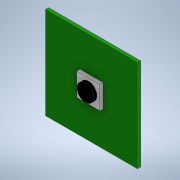
# Autodesk Inventor part: Nav_Camera
Saved by Autodesk Inventor 2020 (Build 240168000, 168)
## iProperties
Created: 2022-01-28
Part Number: Nav_Camera
Material: Generic
Document SubType Name: Modeling
Designer: danie
Density: 1 g/cm^3
Appearance: Default
Author: danie
Autodesk Inventor part; units mm, degrees
ref_plane "YZ Plane" through (0, 0, 0) normal (1, 0, 0) x (0, 1, 0)
ref_plane "XZ Plane" through (0, 0, 0) normal (0, 1, 0) x (-1, 0, 0)
ref_plane "XY Plane" through (0, 0, 0) normal (0, 0, 1) x (1, 0, 0)
sketch "Sketch1" plane through (0, 0, 0) normal (0, 0, 1) x (1, 0, 0)
  line L0 (0, 0) -> (38, 0)
  line L1 (38, 0) -> (38, -38)
  line L2 (38, -38) -> (0, -38)
  line L3 (0, -38) -> (0, 0)
  dimension "d0" = 38
  dimension "d1" = 38
  constraints: 8 end point, 2 parallel, 1 horizontal, 1 perpendicular
  measures "d0" distance of L1.end L2.end
  measures "d1" distance of L0.end L1.end
extrude "Extrusion1" add sketch "Sketch1" along normal blind 1.27
sketch "Sketch2" plane through (0, 0, 1.27) normal (0, 0, 1) x (1, 0, 0)
  line L0 (0, -38) -> (38, -38) construction
  line L1 (0, 0) -> (38, -38) construction
  line L2 (38, -38) -> (38, 0) construction
  line L3 (38, 0) -> (0, -38) construction
  line L4 (14.2571, -14.2571) -> (23.7429, -14.2571)
  line L5 (23.7429, -14.2571) -> (23.7429, -23.7429)
  line L6 (23.7429, -23.7429) -> (14.2571, -23.7429)
  line L7 (14.2571, -23.7429) -> (14.2571, -14.2571)
  line L8 (14.2571, -14.2571) -> (23.7429, -23.7429) construction
  line L9 (23.7429, -14.2571) -> (14.2571, -23.7429) construction
  point P0 (19, -19)
  constraints: 16 end point, 3 midpoint, 2 parallel, 1 horizontal, 1 perpendicular, 1 point on line
extrude "Extrusion2" add sketch "Sketch2" along normal blind 1.27
sketch "Sketch3" plane through (0, 0, 2.54) normal (0, 0, 1) x (1, 0, 0)
  line L0 (23.7429, -14.2571) -> (14.2571, -14.2571) construction
  line L1 (23.7429, -23.7429) -> (23.7429, -14.2571) construction
  line L2 (14.2571, -14.2571) -> (23.7429, -23.7429) construction
  line L3 (14.2571, -14.2571) -> (14.2571, -23.7429) construction
  line L4 (23.7429, -14.2571) -> (14.2571, -23.7429) construction
  circle A0 centre (19, -19) radius 3.4833
  point P0 (0, 0)
  constraints: 4 end point, 1 centre point, 1 midpoint
extrude "Extrusion3" add sketch "Sketch3" along normal blind 1.27
body "Solid1"
